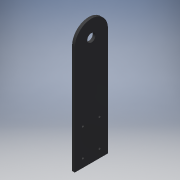
# Autodesk Inventor part: Flipper Plate
Saved by Autodesk Inventor 2017 (Build 210142000, 142)
## iProperties
Created: 2017-01-14
Part Number: Flipper Plate
Material: Generic
Document SubType Name: Modeling
Designer: Ben
Density: 1 g/cm^3
Appearance: Particle Board
Author: Ben
Autodesk Inventor part; units mm, degrees
ref_plane "YZ Plane" through (0, 0, 0) normal (1, 0, 0) x (0, 1, 0)
ref_plane "XZ Plane" through (0, 0, 0) normal (0, 1, 0) x (-1, 0, 0)
ref_plane "XY Plane" through (0, 0, 0) normal (0, 0, 1) x (1, 0, 0)
sketch "Sketch1" plane through (0, 0, 0) normal (1, 0, 0) x (0, 1, 0)
  line L0 (0, 19.05) -> (0, -19.05)
  line L1 (0, -19.05) -> (124.46, -19.05)
  line L2 (0, 19.05) -> (124.46, 19.05)
  circle A0 centre (124.46, 0) radius 4.7625
  line L3 (124.46, 0) -> (0, 0) construction
  arc A1 (124.46, -19.05) -> (124.46, 19.05) centre (124.46, 0) ccw
  line L4 (0, 9.525) -> (41.275, 9.525) construction
  line L5 (41.275, 9.525) -> (41.275, -9.525) construction
  line L6 (41.275, -9.525) -> (0, -9.525) construction
  line L7 (9.525, -9.525) -> (9.525, 9.525) construction
  circle A2 centre (41.275, 9.525) radius 1.27
  circle A3 centre (41.275, -9.525) radius 1.27
  circle A4 centre (9.525, -9.525) radius 1.27
  circle A5 centre (9.525, 9.525) radius 1.27
  dimension "d0" = 9.525
  dimension "d1" = 38.1
  dimension "d2" = 124.46
  dimension "d5" = 19.05
  dimension "d6" = 31.75
  dimension "d7" = 9.525
  dimension "d8" = 2.54
  constraints: 16 end point, 6 centre point, 6 coincident, 5 perpendicular, 4 point on line, 3 equal radius, 2 horizontal, 2 point on circle, 1 midpoint, 1 parallel, 1 tangent, 1 vertical, 1 other
  measures "d0" diameter of A0
  measures "d1" distance of L0.start L0.end
  measures "d2" distance of L3.start L3.end
  measures "d5" distance of L4.end L5.end
  measures "d6" distance between parallel lines of L7 L5
  measures "d7" distance between parallel lines of L0 L7
  measures "d8" diameter of A2
extrude "Extrusion1" add sketch "Sketch1" along normal blind 3.175
body "Solid1"
